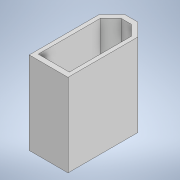
# Autodesk Inventor part: TX60
Saved by Autodesk Inventor 2020 (Build 240168000, 168)
## iProperties
Created: 2020-02-20
Part Number: TX60
Material: Generic
Document SubType Name: Modeling
Designer: atmat
Density: 1 g/cm^3
Appearance: Default
Author: atmat
Autodesk Inventor part; units mm, degrees
ref_plane "YZ Plane" through (0, 0, 0) normal (1, 0, 0) x (0, 1, 0)
ref_plane "XZ Plane" through (0, 0, 0) normal (0, 1, 0) x (-1, 0, 0)
ref_plane "XY Plane" through (0, 0, 0) normal (0, 0, 1) x (1, 0, 0)
sketch "Sketch1" plane through (0, 0, 0) normal (0, 1, 0) x (-1, 0, 0)
  line L0 (3.75, 8) -> (-3.75, 8)
  line L1 (-3.75, 8) -> (-3.75, -5.5)
  line L2 (-3.75, -5.5) -> (-1.25, -8)
  line L3 (-1.25, -8) -> (1.25, -8)
  line L4 (1.25, -8) -> (3.75, -5.5)
  line L5 (3.75, -5.5) -> (3.75, 8)
  point P0 (0, 0)
  dimension "d0" = 7.5
  dimension "d1" = 3.75
  dimension "d2" = 16
  dimension "d3" = 8
  dimension "d4" = 2.5
  dimension "d5" = 135
  dimension "d6" = 135
  constraints: 12 end point, 3 parallel, 1 horizontal, 1 perpendicular
  measures "d0" distance of L0.start L0.end
  measures "d1" distance from line of point (0, 0) L5
  measures "d2" distance between parallel lines of L3 L0
  measures "d3" distance from line of point (0, 0) L0
  measures "d4" distance of L2.end L3.end
  measures "d5" angle of L3 L4
  measures "d6" angle of L3 L2
extrude "Extrusion1" add sketch "Sketch1" along normal blind 16
sketch "Sketch2" plane through (0, 16, 0) normal (0, 1, 0) x (1, 0, 0)
  line L0 (-3, -7) -> (3, -7)
  line L1 (3, -7) -> (3, 5)
  line L2 (3, 5) -> (1, 7)
  line L3 (1, 7) -> (-1, 7)
  line L4 (-1, 7) -> (-3, 5)
  line L5 (-3, 5) -> (-3, -7)
  line L6 (-3.75, 5.5) -> (-3.75, -8) projected
  line L7 (-1.25, 8) -> (-3.75, 5.5) projected
  line L8 (1.25, 8) -> (-1.25, 8) projected
  line L9 (3.75, 5.5) -> (1.25, 8) projected
  point P0 (0, 0)
  dimension "d9" = 14
  dimension "d10" = 2
  dimension "d11" = 7
  dimension "d12" = 6
  dimension "d13" = 3
  constraints: 12 end point, 5 parallel, 2 perpendicular, 1 horizontal
  measures "d9" distance between parallel lines of L3 L0
  measures "d10" distance of L2.end L3.end
  measures "d11" distance from line of point (0, 0) L0
  measures "d12" distance between parallel lines of L1 L5
  measures "d13" distance from line of point (0, 0) L1
extrude "Extrusion2" cut sketch "Sketch2" against normal blind 8
body "Solid1"
